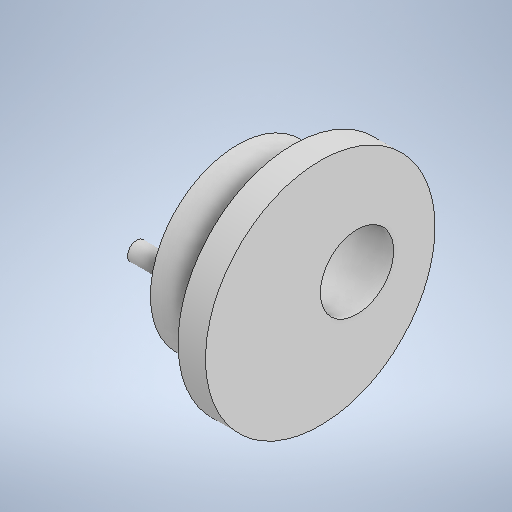
# Autodesk Inventor part: 203
Saved by Autodesk Inventor 2025.1 (Build 291241000, 241)
## iProperties
Created: 2024-08-01
Part Number: 203
Material: Generisch
Document SubType Name: Modeling
Designer: ffogue
Density: 1 g/cm^3
Appearance: Vorgabe
Author: ffogue
Autodesk Inventor part; units mm, degrees
ref_plane "YZ Plane" through (0, 0, 0) normal (1, 0, 0) x (0, 1, 0)
ref_plane "XZ Plane" through (0, 0, 0) normal (0, 1, 0) x (-1, 0, 0)
ref_plane "XY Plane" through (0, 0, 0) normal (0, 0, 1) x (1, 0, 0)
sketch "Sketch1" plane through (0, 0, 0) normal (0, 0, 1) x (1, 0, 0)
  line L0 (0, 0) -> (0, 9.5)
  line L1 (0, 9.5) -> (6, 9.5)
  line L2 (6, 9.5) -> (6, 12.5)
  line L3 (6, 12.5) -> (9, 12.5)
  line L4 (9, 12.5) -> (9, 0)
  line L5 (9, 0) -> (0, 0)
  point P0 (7.5, 12.5)
  dimension "d0" = 3
  dimension "d1" = 6
  dimension "d2" = 25
  dimension "d3" = 19
  constraints: 12 end point, 5 perpendicular, 1 midpoint, 1 vertical
  measures "d0" distance of L2.end L3.end
  measures "d1" distance of L0.end L1.end
  measures "d2" diameter of point (7.5, 12.5) L5
  measures "d3" diameter of L1 L5
revolve "Revolution1" add sketch "Sketch1" angle 360 about axis through (9, 0, 0) along (-1, 0, 0)
sketch "Sketch2" plane through (0, 0, 0) normal (-1, 0, 0) x (0, 0, 1)
  point P0 (0, 0)
  point P1 (0, 4)
  dimension "d12" = 4
  constraints: 1 vertical alignment
  measures "d12" distance of point (0, 0) point (0, 4)
hole "Hole1" at (0, 4, 0) direction (1, 0, 0) diameter 8 depth 9
sketch "Sketch4" plane through (0, 0, 0) normal (-1, 0, 0) x (0, 0, 1)
  circle A0 centre (0, -6) radius 1
  point P0 (0, 0)
  dimension "d21" = 6
  dimension "d22" = 2
  constraints: 1 centre point, 1 vertical alignment
  measures "d21" distance of A0.centre point (0, 0)
  measures "d22" diameter of A0
extrude "Extrusion1" add sketch "Sketch4" along normal blind 5
body "Solid1"
